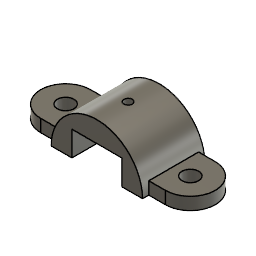
Record 6 (Autodesk Fusion 360 design; units mm, degrees)
part number: 2025-09-30-13-48-39-662
Autodesk Fusion 360 part; units mm, degrees
sketch "Sketch1" plane through (0, 0, 0) normal (0, 0, 1) x (1, 0, 0)
  arc A0 (110, 0) -> (-110, 0) centre (0, 0) ccw
  line L0 (-110, 0) -> (110, 0)
  line L1 (-60, 60) -> (60, 60)
  line L2 (60, 60) -> (60, 0)
  line L3 (60, 0) -> (-60, 0)
  line L4 (-60, 0) -> (-60, 60)
  dimension "d1" = 220
  dimension "d4" = 120
  dimension "d5" = 60
  constraint coincident A0.centre origin
  constraint horizontal L1
  constraint vertical L2
  constraint horizontal L3
  constraint vertical L4
  measures "d1" diameter of A0
  measures "d4" distance of L1.start L1.end
  measures "d5" distance of A0.centre L2
extrude "Extrude1" add sketch "Sketch1" along normal blind 150 contours A0 L0 L1 L2 L4 makes body 1
sketch "Sketch2" plane through (0, 60, 0) normal (0, -1, 0) x (1, 0, 0)
  line L0 (-60, 0) -> (60, 0)
  line L1 (60, 0) -> (60, 150)
  line L2 (60, 150) -> (-60, 150)
  line L3 (-60, 150) -> (-60, 0)
  circle A0 centre (150, 75) radius 20
  line L4 (0, -50) -> (0, 0)
  line L5 (0, 150) -> (0, 180)
  arc A1 (150, 15) -> (150, 135) centre (150, 75) ccw
  line L6 (150, 135) -> (110, 135)
  line L7 (150, 15) -> (110, 15)
  line L8 (0, -60) -> (0, 194.892)
  arc A2 (-150, 135) -> (-150, 15) centre (-150, 75) ccw
  circle A3 centre (-150, 75) radius 20
  line L9 (-150, 135) -> (-110, 135)
  line L10 (-150, 15) -> (-110, 15)
  line L11 (110, 15) -> (110, 135)
  line L12 (-110, 15) -> (-110, 135)
  constraint perpendicular L2 L4
  constraint coincident L0 L4.end
  constraint coincident L2 L5.start
  constraint collinear L4 L5
  constraint tangent A1 L6
  constraint horizontal L6
  constraint tangent A1 L7
  constraint parallel L6 L7
  constraint perpendicular L2 L8
  constraint symmetric A0 L8 A3
  constraint symmetric A1 L8 A2
  constraint symmetric A1.end L8 A2.start
  constraint symmetric L6.end L8 L9.end
  constraint symmetric A1.start L8 A2.end
  constraint symmetric L7.end L8 L10.end
  constraint perpendicular L6 L11
extrude "Extrude2" add sketch "Sketch2" along normal blind 60 separate body contours A1 L6 L7 L11 | A2 L9 L10 L12 makes body 2 at (161.8888, 20, 133.8103) makes body 3 at (-161.8888, 20, 16.1897)
extrude "Extrude3" cut 2 faces at (134.2311, 60, 28.7942) (-134.2311, 60, 28.7942) along direction (0, -1, 0) blind 30 on bodies 2 3 bodies 2 3
combine "Combine1" operation add target body 1 tool bodies 2 3
sketch "Sketch3" plane through (0, 60, 0) normal (0, -1, 0) x (1, 0, 0)
  line L0 (-60, 0) -> (60, 0)
  line L1 (60, 0) -> (60, 150)
  line L2 (60, 150) -> (-60, 150)
  line L3 (-60, 150) -> (-60, 0)
  circle A0 centre (0, 75) radius 10
  dimension "d16" = 20
  dimension "d17" = 75
  measures "d16" diameter of A0
  measures "d17" distance of origin A0.centre
extrude "Extrude4" cut sketch "Sketch3" along normal mid plane 200 contours A0 bodies 1
sketch "Sketch4" plane through (0, 0, 0) normal (0, 0, 1) x (1, 0, 0)
